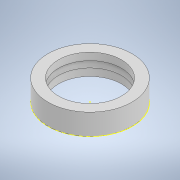
# Autodesk Inventor part: Bearing
Saved by Autodesk Inventor 2020.3 (Build 243373000, 373)
## iProperties
Created: 2020-08-08
Part Number: Bearing
Material: Generic
Document SubType Name: Modeling
Designer: joesp
Density: 1 g/cm^3
Appearance: Default
Author: joesp
Autodesk Inventor part; units mm, degrees
ref_plane "YZ Plane" through (0, 0, 0) normal (1, 0, 0) x (0, 1, 0)
ref_plane "XZ Plane" through (0, 0, 0) normal (0, 1, 0) x (-1, 0, 0)
ref_plane "XY Plane" through (0, 0, 0) normal (0, 0, 1) x (1, 0, 0)
sketch "Sketch2" plane through (0, 0, 0) normal (1, 0, 0) x (0, 1, 0)
  line L0 (0, -15) -> (10, -15)
  line L1 (10, -15) -> (10, -20)
  line L2 (10, -20) -> (0, -20)
  line L3 (0, -20) -> (0, -15)
  line L4 (0, 0) -> (10, 0) construction
  line L5 (10, 0) -> (10, -10.5) construction
  line L6 (10, -10.5) -> (0, -10.5) construction
  line L7 (0, -10.5) -> (0, 0) construction
  circle A0 centre (5, -13) radius 2.5
  point P0 (5, -15)
  point P1 (6.5, -15)
  point P2 (3.5, -15)
  dimension "d5" = 15
  dimension "d6" = 5
  dimension "d7" = 10
  dimension "d8" = 10.5
  dimension "d9" = 5
  constraints: 16 end point, 4 parallel, 2 horizontal, 2 perpendicular, 2 point on circle, 2 point on line, 2 vertical alignment, 1 centre point, 1 collinear, 1 midpoint, 1 tangent
  measures "d5" distance from line of L4.start L0
  measures "d6" distance of L0.end L1.end
  measures "d7" distance of L1.end L2.end
  measures "d8" distance of L4.end L5.end
  measures "d9" diameter of A0
revolve "Revolution1" add sketch "Sketch2" angle 360 about axis through (0, 0, 0) along (0, 1, 0) contours L0 A0 L1 L2 L3
sketch "Sketch3" plane through (0, 0, 0) normal (0, 1, 0) x (-1, 0, 0)
  circle A0 centre (0, 0) radius 20 projected
  circle A1 centre (0, 0) radius 20 projected
body "Solid2"
